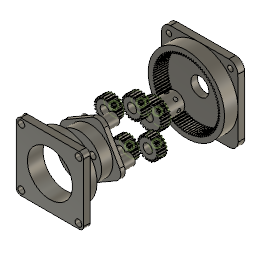
Planetary gear box (simple) (Autodesk Fusion 360 design; units mm, degrees)
part number: 2026-04-07-13-28-31-820
part number: 2026-04-07-13-34-58-780
part number: 2026-04-07-13-35-47-978
part number: 2026-04-07-13-42-23-134
description: Spur Gear; Module: 2.0; Num Teeth: 22; Pressure Angle: 20.0; Backlash: 0.00 mm
part number: 2026-04-07-13-45-37-239
part number: 2026-04-07-13-52-50-834
description: Spur Gear; Module: 2.0; Num Teeth: 28; Pressure Angle: 20.0; Backlash: 0.00 mm
part number: 2026-04-07-13-54-13-736
description: Spur Gear; Module: 1.6; Num Teeth: 88; Pressure Angle: 20.0; Backlash: 0.00 mm
part number: 2026-04-07-14-14-13-761
part number: 2026-04-07-14-24-32-311
Autodesk Fusion 360 part; units mm, degrees
(part 1 of 15)
sketch "Sketch1" plane through (0, 0, 0) normal (0, 1, 0) x (1, 0, 0)
  line L0 (65, -75) -> (-65, -75)
  line L1 (-75, -65) -> (-75, 65)
  line L2 (-65, 75) -> (65, 75)
  line L3 (75, 65) -> (75, -65)
  line L4 (75, -75) -> (-75, 75) construction
  line L5 (-75, -75) -> (75, 75) construction
  circle A0 centre (0, 0) radius 50
  circle A1 centre (63.6396, -63.6396) radius 7.5
  circle A2 centre (-63.6396, -63.6396) radius 7.5
  circle A3 centre (-63.6396, 63.6396) radius 7.5
  circle A4 centre (63.6396, 63.6396) radius 7.5
  arc A5 (65, -75) -> (75, -65) centre (65, -65) ccw
  arc A6 (-75, -65) -> (-65, -75) centre (-65, -65) ccw
  arc A7 (-65, 75) -> (-75, 65) centre (-65, 65) ccw
  arc A8 (75, 65) -> (65, 75) centre (65, 65) ccw
  dimension "d1" = 150
  dimension "d2" = 150
  dimension "d3" = 100
  dimension "d4" = 15
  dimension "d5" = 90
  dimension "d6" = 15
  dimension "d7" = 90
  dimension "d8" = 15
  dimension "d9" = 15
  dimension "d10" = 90
  dimension "d11" = 90
  dimension "d12" = 10
  constraint horizontal L0
  constraint perpendicular L0 L1
  constraint parallel L0 L2
  constraint parallel L1 L3
  constraint coincident L4 A0.centre
  constraint coincident L5 A0.centre
  constraint coincident A0.centre origin
  constraint coincident L4 A1.centre
  constraint coincident L5 A2.centre
  constraint coincident L4 A3.centre
  constraint coincident L5 A4.centre
  constraint coincident L4.start L3
  constraint coincident L4.start L0
  constraint tangent L3 A5
  constraint tangent L0 A5
  constraint coincident L5.start L0
  constraint coincident L5.start L1
  constraint tangent L0 A6
  constraint tangent L1 A6
  constraint equal A5 A6
  constraint coincident L4.end L2
  constraint coincident L4.end L1
  constraint tangent L2 A7
  constraint tangent L1 A7
  constraint equal A5 A7
  constraint coincident L5.end L2
  constraint coincident L5.end L3
  constraint tangent L2 A8
  constraint tangent L3 A8
  constraint equal A5 A8
  measures "d1" distance of L4.end L5.end
  measures "d2" distance of L5.start L4.end
  measures "d3" diameter of A0
  measures "d4" diameter of A1
  measures "d5" distance of A0.centre A1.centre
  measures "d6" diameter of A2
  measures "d7" distance of A0.centre A2.centre
  measures "d8" diameter of A4
  measures "d9" diameter of A3
  measures "d10" distance of A0.centre A4.centre
  measures "d11" distance of A0.centre A3.centre
  measures "d12" radius of A5
extrude "Extrude1" add sketch "Sketch1" along normal blind 15 makes body 1
sketch "Sketch2" plane through (0, 15, 0) normal (0, 1, 0) x (-1, 0, 0)
  circle A0 centre (0, 0) radius 50
  circle A1 centre (63.6396, -63.6396) radius 7.5
  circle A2 centre (-63.6396, 63.6396) radius 7.5
  circle A3 centre (-63.6396, -63.6396) radius 7.5
  circle A4 centre (63.6396, 63.6396) radius 7.5
  arc A5 (-65, 75) -> (-75, 65) centre (-65, 65) ccw
  line L0 (-75, 65) -> (-75, -65)
  arc A6 (-75, -65) -> (-65, -75) centre (-65, -65) ccw
  line L1 (-65, -75) -> (65, -75)
  arc A7 (65, -75) -> (75, -65) centre (65, -65) ccw
  line L2 (75, -65) -> (75, 65)
  arc A8 (75, 65) -> (65, 75) centre (65, 65) ccw
  line L3 (65, 75) -> (-65, 75)
  circle A9 centre (0, 0) radius 70
  dimension "d15" = 140
  constraint coincident A0.centre A9.centre
  measures "d15" diameter of A9
extrude "Extrude2" add sketch "Sketch2" along normal blind 20 contours A9 bodies 1
ref_plane "WorkPlane1" through (0, 65, 0) normal (0, 1, 0) x (-1, 0, 0)
copy_body "Body->Comp1" bodies 1 removing the originals makes body 2 in component "Component"
sketch "Sketch1 (2)" plane through (0, 65, 0) normal (0, 1, 0) x (1, 0, 0) in component "planet gear holder"
  circle A0 centre (0, 0) radius 50
  circle A1 centre (0, 0) radius 50
  line L0 (35, 55) -> (-35, 55)
  line L1 (-55, 35) -> (-55, -35)
  line L2 (-35, -55) -> (35, -55)
  line L3 (55, -35) -> (55, 35)
  line L4 (55, 55) -> (-55, -55) construction
  line L5 (-55, 55) -> (55, -55) construction
  line L6 (0, -50) -> (0, 50) construction
  circle A2 centre (0, -35) radius 7.5
  circle A3 centre (35, 0) radius 7.5
  circle A4 centre (0, 35) radius 7.5
  circle A5 centre (-35, 0) radius 7.5
  arc A6 (35, -55) -> (55, -35) centre (35, -35) ccw
  arc A7 (55, 35) -> (35, 55) centre (35, 35) ccw
  arc A8 (-35, 55) -> (-55, 35) centre (-35, 35) ccw
  arc A9 (-55, -35) -> (-35, -55) centre (-35, -35) ccw
  circle A10 centre (35, -35) radius 12.5
  circle A11 centre (-35, -35) radius 12.5
  circle A12 centre (35, 35) radius 12.5
  circle A13 centre (-35, 35) radius 12.5
  dimension "d19" = 110
  dimension "d20" = 110
  dimension "d21" = 15
  dimension "d22" = 35
  dimension "d24" = 360
  dimension "d25" = 20
  dimension "d28" = 25
  dimension "d29" = 25
  dimension "d30" = 25
  dimension "d31" = 25
  constraint concentric A0 A1
  constraint horizontal L0
  constraint perpendicular L0 L1
  constraint parallel L0 L2
  constraint parallel L1 L3
  constraint coincident L4 A0.centre
  constraint coincident L5 A0.centre
  constraint coincident A0.centre A1.centre
  constraint coincident A0 L6.start
  constraint coincident A1 L6.end
  constraint vertical L6
  constraint coincident L6 A2.centre
  constraint coincident L5.end L2
  constraint coincident L5.end L3
  constraint tangent L2 A6
  constraint tangent L3 A6
  constraint coincident L4.start L3
  constraint coincident L4.start L0
  constraint tangent L3 A7
  constraint tangent L0 A7
  constraint equal A6 A7
  constraint coincident L5.start L0
  constraint coincident L5.start L1
  constraint tangent L0 A8
  constraint tangent L1 A8
  constraint equal A6 A8
  constraint coincident L4.end L2
  constraint coincident L4.end L1
  constraint tangent L2 A9
  constraint tangent L1 A9
  constraint equal A6 A9
  constraint concentric A6 A10
  constraint concentric A9 A11
  constraint concentric A7 A12
  constraint concentric A8 A13
  measures "d19" distance of L4.end L5.end
  measures "d20" distance of L5.start L4.end
  measures "d21" diameter of A2
  measures "d22" distance of A0.centre A2.centre
  measures "d25" radius of A6
  measures "d28" diameter of A10
  measures "d29" diameter of A11
  measures "d30" diameter of A12
  measures "d31" diameter of A13
extrude "Extrude1'" add sketch "Sketch1 (2)" against normal blind 25 separate body contours A0 A1 A10 A11 A12 A13 | A0 A1 A12 | A0 A1 A10 | A0 A1 A13 | A0 A1 A11 picked at (29.7361, 35.2337) picked at (29.7361, -35.2337) picked at (-35.4165, 29.6761) picked at (-35.4165, -29.6761) makes body 3 in component "planet gear holder"
extrude "Extrude2'" add sketch "Sketch1 (2)" along normal blind 40 separate body contours A0 A1 A12 | A0 A1 A12 | A0 A1 A10 | A0 A1 A10 | A0 A1 A13 | A0 A1 A13 | A0 A1 A11 | A0 A1 A11 makes body 4 at (47.4379, 91.6667, -36.2446) makes body 5 at (-22.5621, 91.6667, -36.2446) makes body 6 at (47.4379, 91.6667, 33.7554) makes body 7 at (-22.5621, 78.3333, 36.2446) in component "planet gear holder"
extrude "Extrude3" add sketch "Sketch1 (2)" along normal blind 10 contours A0 A1 A10 A11 A12 A13 | L0 L1 L2 L3 A6 A7 A8 A9 bodies 3 4 5 6 7 in component "planet gear holder"
sketch "Base Circle" plane through (0, 0, 0) normal (0, 0, 1) x (1, 0, 0) in component "Spur Gear 22 teeth"
  circle A0 centre (0, 0) radius 19.686
  circle A1 centre (0, 0) radius 10
extrude "Extrude1''" add sketch "Base Circle" along normal blind 20 separate body makes body 8 in component "Spur Gear 22 teeth"
sketch "Gear Tooth" plane through (0, 0, 0) normal (0, 0, 1) x (1, 0, 0) in component "Spur Gear 22 teeth"
  spline S0 degree 5 poles (20.5963, -1.782) (20.606, -1.7828) (20.6255, -1.7842) (20.6547, -1.7856) (20.6937, -1.7861) (20.7426, -1.7846) (20.7915, -1.7818) (20.8404, -1.7781) (20.8894, -1.7739) (20.9384, -1.7693) (20.9874, -1.7645) (21.0364, -1.7592) (21.0854, -1.7533) (21.1344, -1.7468) (21.1835, -1.7395) (21.2325, -1.7317) (21.2815, -1.7232) (21.3306, -1.7143) (21.3796, -1.705) (21.4286, -1.6954) (21.4776, -1.6853) (21.5266, -1.6749) (21.5756, -1.6641) (21.6246, -1.6528) (21.6736, -1.6411) (21.7225, -1.629) (21.7714, -1.6165) (21.8204, -1.6036) (21.8693, -1.5904) (21.9182, -1.5768) (21.967, -1.5629) (22.0159, -1.5487) (22.0647, -1.5341) (22.1135, -1.5191) (22.1622, -1.5038) (22.211, -1.4882) (22.2597, -1.4723) (22.3084, -1.456) (22.3571, -1.4394) (22.4057, -1.4225) (22.4543, -1.4053) (22.5029, -1.3878) (22.5514, -1.37) (22.6, -1.3519) (22.6484, -1.3335) (22.6969, -1.3148) (22.7453, -1.2958) (22.7937, -1.2765) (22.842, -1.2569) (22.8903, -1.237) (22.9386, -1.2169) (22.9868, -1.1964) (23.035, -1.1757) (23.0832, -1.1548) (23.1313, -1.1335) (23.1794, -1.112) (23.2274, -1.0902) (23.2754, -1.0681) (23.3233, -1.0457) (23.3712, -1.0231) (23.4191, -1.0003) (23.4669, -0.9772) (23.5146, -0.9538) (23.5624, -0.9301) (23.61, -0.9062) (23.6577, -0.8821) (23.7052, -0.8577) (23.7528, -0.833) (23.8002, -0.8081) (23.8477, -0.7829) (23.895, -0.7575) (23.9329, -0.737) (23.9613, -0.7215) (23.9802, -0.7111) (23.9896, -0.7059) knots 0 0 0 0 0 0 0.01428571 0.02857143 0.04285714 0.05714286 0.07142857 0.08571429 0.1 0.11428571 0.12857143 0.14285714 0.15714286 0.17142857 0.18571429 0.2 0.21428571 0.22857143 0.24285714 0.25714286 0.27142857 0.28571429 0.3 0.31428571 0.32857143 0.34285714 0.35714286 0.37142857 0.38571429 0.4 0.41428571 0.42857143 0.44285714 0.45714286 0.47142857 0.48571429 0.5 0.51428571 0.52857143 0.54285714 0.55714286 0.57142857 0.58571429 0.6 0.61428571 0.62857143 0.64285714 0.65714286 0.67142857 0.68571429 0.7 0.71428571 0.72857143 0.74285714 0.75714286 0.77142857 0.78571429 0.8 0.81428571 0.82857143 0.84285714 0.85714286 0.87142857 0.88571429 0.9 0.91428571 0.92857143 0.94285714 0.95714286 0.97142857 0.98571429 1 1 1 1 1 1
  spline S1 degree 5 poles (20.5963, 1.782) (20.606, 1.7828) (20.6255, 1.7842) (20.6547, 1.7856) (20.6937, 1.7861) (20.7426, 1.7846) (20.7915, 1.7818) (20.8404, 1.7781) (20.8894, 1.7739) (20.9384, 1.7693) (20.9874, 1.7645) (21.0364, 1.7592) (21.0854, 1.7533) (21.1344, 1.7468) (21.1835, 1.7395) (21.2325, 1.7317) (21.2815, 1.7232) (21.3306, 1.7143) (21.3796, 1.705) (21.4286, 1.6954) (21.4776, 1.6853) (21.5266, 1.6749) (21.5756, 1.6641) (21.6246, 1.6528) (21.6736, 1.6411) (21.7225, 1.629) (21.7714, 1.6165) (21.8204, 1.6036) (21.8693, 1.5904) (21.9182, 1.5768) (21.967, 1.5629) (22.0159, 1.5487) (22.0647, 1.5341) (22.1135, 1.5191) (22.1622, 1.5038) (22.211, 1.4882) (22.2597, 1.4723) (22.3084, 1.456) (22.3571, 1.4394) (22.4057, 1.4225) (22.4543, 1.4053) (22.5029, 1.3878) (22.5514, 1.37) (22.6, 1.3519) (22.6484, 1.3335) (22.6969, 1.3148) (22.7453, 1.2958) (22.7937, 1.2765) (22.842, 1.2569) (22.8903, 1.237) (22.9386, 1.2169) (22.9868, 1.1964) (23.035, 1.1757) (23.0832, 1.1548) (23.1313, 1.1335) (23.1794, 1.112) (23.2274, 1.0902) (23.2754, 1.0681) (23.3233, 1.0457) (23.3712, 1.0231) (23.4191, 1.0003) (23.4669, 0.9772) (23.5146, 0.9538) (23.5624, 0.9301) (23.61, 0.9062) (23.6577, 0.8821) (23.7052, 0.8577) (23.7528, 0.833) (23.8002, 0.8081) (23.8477, 0.7829) (23.895, 0.7575) (23.9329, 0.737) (23.9613, 0.7215) (23.9802, 0.7111) (23.9896, 0.7059) knots 0 0 0 0 0 0 0.01428571 0.02857143 0.04285714 0.05714286 0.07142857 0.08571429 0.1 0.11428571 0.12857143 0.14285714 0.15714286 0.17142857 0.18571429 0.2 0.21428571 0.22857143 0.24285714 0.25714286 0.27142857 0.28571429 0.3 0.31428571 0.32857143 0.34285714 0.35714286 0.37142857 0.38571429 0.4 0.41428571 0.42857143 0.44285714 0.45714286 0.47142857 0.48571429 0.5 0.51428571 0.52857143 0.54285714 0.55714286 0.57142857 0.58571429 0.6 0.61428571 0.62857143 0.64285714 0.65714286 0.67142857 0.68571429 0.7 0.71428571 0.72857143 0.74285714 0.75714286 0.77142857 0.78571429 0.8 0.81428571 0.82857143 0.84285714 0.85714286 0.87142857 0.88571429 0.9 0.91428571 0.92857143 0.94285714 0.95714286 0.97142857 0.98571429 1 1 1 1 1 1
  arc A0 (23.9896, -0.7059) -> (23.9896, 0.7059) centre (0, 0) ccw
  line L0 (19.6028, -1.696) -> (20.5963, -1.782)
  line L1 (19.6028, 1.696) -> (20.5963, 1.782)
  line L2 (19.6028, -1.696) -> (19.6028, 1.696)
  point P0 (20.8351, -1.7784)
  point P1 (21.0756, -1.7544)
  point P2 (21.3171, -1.7167)
  point P3 (21.5593, -1.6676)
  point P4 (21.8021, -1.6084)
  point P5 (22.0453, -1.5398)
  point P6 (22.2887, -1.4626)
  point P7 (22.5322, -1.377)
  point P8 (22.7757, -1.2836)
  point P9 (23.0191, -1.1825)
  point P10 (23.2623, -1.074)
  point P11 (23.5052, -0.9583)
  point P12 (23.7477, -0.8356)
  point P13 (20.8351, 1.7784)
  point P14 (21.0756, 1.7544)
  point P15 (21.3171, 1.7167)
  point P16 (21.5593, 1.6676)
  point P17 (21.8021, 1.6084)
  point P18 (22.0453, 1.5398)
  point P19 (22.2887, 1.4626)
  point P20 (22.5322, 1.377)
  point P21 (22.7757, 1.2836)
  point P22 (23.0191, 1.1825)
  point P23 (23.2623, 1.074)
  point P24 (23.5052, 0.9583)
  point P25 (23.7477, 0.8356)
extrude "Extrude2''" add sketch "Gear Tooth" along normal blind 20 bodies 8 in component "Spur Gear 22 teeth"
pattern_circular "C-Pattern1" count 22 over 360 about axis through (0, 0, 0) along (0, 0, 1) of "Extrude2''" in component "Spur Gear 22 teeth"
sketch "Diametrial Pitch Circle" plane through (0, 0, 0) normal (0, 0, 1) x (1, 0, 0) in component "Spur Gear 22 teeth"
  circle A0 centre (0, 0) radius 22 construction
sketch "Base Circle (2)" plane through (0, 0, 0) normal (0, 0, 1) x (1, 0, 0) in component "Spur Gear 28 teeth"
  circle A0 centre (0, 0) radius 25.686
  circle A1 centre (0, 0) radius 10
extrude "Extrude1'''" add sketch "Base Circle (2)" along normal blind 20 separate body makes body 9 in component "Spur Gear 28 teeth"
sketch "Gear Tooth (2)" plane through (0, 0, 0) normal (0, 0, 1) x (1, 0, 0) in component "Spur Gear 28 teeth"
  spline S0 degree 5 poles (26.2451, -1.8667) (26.2559, -1.8674) (26.2774, -1.8687) (26.3098, -1.8698) (26.3529, -1.8699) (26.4069, -1.8679) (26.461, -1.8644) (26.515, -1.8601) (26.5691, -1.8552) (26.6232, -1.8501) (26.6773, -1.8446) (26.7314, -1.8386) (26.7855, -1.8321) (26.8396, -1.8248) (26.8937, -1.8169) (26.9478, -1.8082) (27.0019, -1.7991) (27.056, -1.7894) (27.1101, -1.7794) (27.1642, -1.7689) (27.2182, -1.7581) (27.2723, -1.7469) (27.3263, -1.7352) (27.3803, -1.7231) (27.4343, -1.7106) (27.4883, -1.6977) (27.5423, -1.6844) (27.5962, -1.6707) (27.6502, -1.6566) (27.7041, -1.6422) (27.7579, -1.6274) (27.8118, -1.6123) (27.8656, -1.5968) (27.9194, -1.581) (27.9732, -1.5648) (28.027, -1.5483) (28.0807, -1.5315) (28.1344, -1.5143) (28.1881, -1.4969) (28.2417, -1.4791) (28.2953, -1.461) (28.3489, -1.4425) (28.4025, -1.4238) (28.456, -1.4048) (28.5095, -1.3854) (28.5629, -1.3658) (28.6163, -1.3459) (28.6697, -1.3256) (28.7231, -1.3051) (28.7764, -1.2843) (28.8296, -1.2632) (28.8829, -1.2418) (28.9361, -1.2202) (28.9892, -1.1983) (29.0423, -1.176) (29.0954, -1.1536) (29.1485, -1.1308) (29.2015, -1.1078) (29.2544, -1.0845) (29.3073, -1.0609) (29.3602, -1.0371) (29.413, -1.013) (29.4658, -0.9886) (29.5186, -0.964) (29.5712, -0.9391) (29.6239, -0.914) (29.6765, -0.8886) (29.729, -0.863) (29.7816, -0.8371) (29.834, -0.8109) (29.8864, -0.7845) (29.9283, -0.7632) (29.9597, -0.7471) (29.9806, -0.7364) (29.9911, -0.731) knots 0 0 0 0 0 0 0.01428571 0.02857143 0.04285714 0.05714286 0.07142857 0.08571429 0.1 0.11428571 0.12857143 0.14285714 0.15714286 0.17142857 0.18571429 0.2 0.21428571 0.22857143 0.24285714 0.25714286 0.27142857 0.28571429 0.3 0.31428571 0.32857143 0.34285714 0.35714286 0.37142857 0.38571429 0.4 0.41428571 0.42857143 0.44285714 0.45714286 0.47142857 0.48571429 0.5 0.51428571 0.52857143 0.54285714 0.55714286 0.57142857 0.58571429 0.6 0.61428571 0.62857143 0.64285714 0.65714286 0.67142857 0.68571429 0.7 0.71428571 0.72857143 0.74285714 0.75714286 0.77142857 0.78571429 0.8 0.81428571 0.82857143 0.84285714 0.85714286 0.87142857 0.88571429 0.9 0.91428571 0.92857143 0.94285714 0.95714286 0.97142857 0.98571429 1 1 1 1 1 1
  spline S1 degree 5 poles (26.2451, 1.8667) (26.2559, 1.8674) (26.2774, 1.8687) (26.3098, 1.8698) (26.3529, 1.8699) (26.4069, 1.8679) (26.461, 1.8644) (26.515, 1.8601) (26.5691, 1.8552) (26.6232, 1.8501) (26.6773, 1.8446) (26.7314, 1.8386) (26.7855, 1.8321) (26.8396, 1.8248) (26.8937, 1.8169) (26.9478, 1.8082) (27.0019, 1.7991) (27.056, 1.7894) (27.1101, 1.7794) (27.1642, 1.7689) (27.2182, 1.7581) (27.2723, 1.7469) (27.3263, 1.7352) (27.3803, 1.7231) (27.4343, 1.7106) (27.4883, 1.6977) (27.5423, 1.6844) (27.5962, 1.6707) (27.6502, 1.6566) (27.7041, 1.6422) (27.7579, 1.6274) (27.8118, 1.6123) (27.8656, 1.5968) (27.9194, 1.581) (27.9732, 1.5648) (28.027, 1.5483) (28.0807, 1.5315) (28.1344, 1.5143) (28.1881, 1.4969) (28.2417, 1.4791) (28.2953, 1.461) (28.3489, 1.4425) (28.4025, 1.4238) (28.456, 1.4048) (28.5095, 1.3854) (28.5629, 1.3658) (28.6163, 1.3459) (28.6697, 1.3256) (28.7231, 1.3051) (28.7764, 1.2843) (28.8296, 1.2632) (28.8829, 1.2418) (28.9361, 1.2202) (28.9892, 1.1983) (29.0423, 1.176) (29.0954, 1.1536) (29.1485, 1.1308) (29.2015, 1.1078) (29.2544, 1.0845) (29.3073, 1.0609) (29.3602, 1.0371) (29.413, 1.013) (29.4658, 0.9886) (29.5186, 0.964) (29.5712, 0.9391) (29.6239, 0.914) (29.6765, 0.8886) (29.729, 0.863) (29.7816, 0.8371) (29.834, 0.8109) (29.8864, 0.7845) (29.9283, 0.7632) (29.9597, 0.7471) (29.9806, 0.7364) (29.9911, 0.731) knots 0 0 0 0 0 0 0.01428571 0.02857143 0.04285714 0.05714286 0.07142857 0.08571429 0.1 0.11428571 0.12857143 0.14285714 0.15714286 0.17142857 0.18571429 0.2 0.21428571 0.22857143 0.24285714 0.25714286 0.27142857 0.28571429 0.3 0.31428571 0.32857143 0.34285714 0.35714286 0.37142857 0.38571429 0.4 0.41428571 0.42857143 0.44285714 0.45714286 0.47142857 0.48571429 0.5 0.51428571 0.52857143 0.54285714 0.55714286 0.57142857 0.58571429 0.6 0.61428571 0.62857143 0.64285714 0.65714286 0.67142857 0.68571429 0.7 0.71428571 0.72857143 0.74285714 0.75714286 0.77142857 0.78571429 0.8 0.81428571 0.82857143 0.84285714 0.85714286 0.87142857 0.88571429 0.9 0.91428571 0.92857143 0.94285714 0.95714286 0.97142857 0.98571429 1 1 1 1 1 1
  arc A0 (29.9911, -0.731) -> (29.9911, 0.731) centre (0, 0) ccw
  line L0 (25.6113, -1.8216) -> (26.2451, -1.8667)
  line L1 (25.6113, 1.8216) -> (26.2451, 1.8667)
  line L2 (25.6113, -1.8216) -> (25.6113, 1.8216)
  point P0 (26.5097, -1.8604)
  point P1 (26.7757, -1.8331)
  point P2 (27.0425, -1.7918)
  point P3 (27.31, -1.7387)
  point P4 (27.5779, -1.6753)
  point P5 (27.8462, -1.6024)
  point P6 (28.1146, -1.5206)
  point P7 (28.3831, -1.4305)
  point P8 (28.6517, -1.3324)
  point P9 (28.9201, -1.2266)
  point P10 (29.1884, -1.1134)
  point P11 (29.4563, -0.9929)
  point P12 (29.7239, -0.8654)
  point P13 (26.5097, 1.8604)
  point P14 (26.7757, 1.8331)
  point P15 (27.0425, 1.7918)
  point P16 (27.31, 1.7387)
  point P17 (27.5779, 1.6753)
  point P18 (27.8462, 1.6024)
  point P19 (28.1146, 1.5206)
  point P20 (28.3831, 1.4305)
  point P21 (28.6517, 1.3324)
  point P22 (28.9201, 1.2266)
  point P23 (29.1884, 1.1134)
  point P24 (29.4563, 0.9929)
  point P25 (29.7239, 0.8654)
extrude "Extrude2'''" add sketch "Gear Tooth (2)" along normal blind 20 bodies 9 in component "Spur Gear 28 teeth"
pattern_circular "C-Pattern1'" count 28 over 360 about axis through (0, 0, 0) along (0, 0, 1) of "Extrude2'''" in component "Spur Gear 28 teeth"
sketch "Diametrial Pitch Circle (2)" plane through (0, 0, 0) normal (0, 0, 1) x (1, 0, 0) in component "Spur Gear 28 teeth"
  circle A0 centre (0, 0) radius 28 construction
sketch "Sketch4" plane through (0, 0, 0) normal (0, 0, -1) x (1, 0, 0) in component "Spur Gear 28 teeth"
  circle A0 centre (0, 0) radius 10
  arc A1 (24.5734, 7.4779) -> (23.8746, 9.4748) centre (0, 0) ccw
  line L0 (23.8746, 9.4748) -> (24.4559, 9.7055)
  spline S0 degree 5 poles (24.4559, 9.7055) (24.466, 9.7095) (24.4859, 9.7177) (24.5156, 9.7307) (24.5545, 9.7494) (24.6023, 9.7746) (24.6494, 9.8012) (24.6963, 9.8286) (24.7429, 9.8564) (24.7894, 9.8845) (24.8357, 9.9129) (24.8819, 9.9418) (24.9278, 9.9712) (24.9734, 10.0012) (25.0187, 10.0318) (25.0637, 10.0631) (25.1085, 10.0948) (25.153, 10.127) (25.1974, 10.1595) (25.2416, 10.1924) (25.2856, 10.2256) (25.3294, 10.2591) (25.3731, 10.2931) (25.4165, 10.3274) (25.4597, 10.3621) (25.5027, 10.3972) (25.5456, 10.4326) (25.5882, 10.4683) (25.6307, 10.5044) (25.673, 10.5408) (25.7151, 10.5775) (25.7571, 10.6145) (25.7989, 10.6518) (25.8405, 10.6894) (25.882, 10.7273) (25.9232, 10.7654) (25.9643, 10.8039) (26.0053, 10.8427) (26.0461, 10.8817) (26.0867, 10.921) (26.1271, 10.9606) (26.1674, 11.0004) (26.2075, 11.0406) (26.2475, 11.0809) (26.2873, 11.1216) (26.3269, 11.1624) (26.3664, 11.2036) (26.4057, 11.245) (26.4449, 11.2866) (26.4839, 11.3285) (26.5227, 11.3706) (26.5614, 11.4129) (26.5999, 11.4555) (26.6383, 11.4984) (26.6765, 11.5414) (26.7146, 11.5847) (26.7525, 11.6282) (26.7902, 11.672) (26.8279, 11.716) (26.8653, 11.7601) (26.9026, 11.8046) (26.9397, 11.8492) (26.9767, 11.894) (27.0136, 11.9391) (27.0502, 11.9844) (27.0868, 12.0299) (27.1231, 12.0755) (27.1594, 12.1215) (27.1954, 12.1676) (27.2314, 12.2139) (27.2671, 12.2604) (27.2956, 12.2978) (27.3169, 12.3259) (27.3311, 12.3447) (27.3382, 12.3541) knots 0 0 0 0 0 0 0.01428571 0.02857143 0.04285714 0.05714286 0.07142857 0.08571429 0.1 0.11428571 0.12857143 0.14285714 0.15714286 0.17142857 0.18571429 0.2 0.21428571 0.22857143 0.24285714 0.25714286 0.27142857 0.28571429 0.3 0.31428571 0.32857143 0.34285714 0.35714286 0.37142857 0.38571429 0.4 0.41428571 0.42857143 0.44285714 0.45714286 0.47142857 0.48571429 0.5 0.51428571 0.52857143 0.54285714 0.55714286 0.57142857 0.58571429 0.6 0.61428571 0.62857143 0.64285714 0.65714286 0.67142857 0.68571429 0.7 0.71428571 0.72857143 0.74285714 0.75714286 0.77142857 0.78571429 0.8 0.81428571 0.82857143 0.84285714 0.85714286 0.87142857 0.88571429 0.9 0.91428571 0.92857143 0.94285714 0.95714286 0.97142857 0.98571429 1 1 1 1 1 1
  arc A2 (27.3382, 12.3541) -> (26.7039, 13.6712) centre (0, 0) ccw
  spline S1 degree 5 poles (22.8361, 13.0691) (22.8455, 13.0745) (22.8643, 13.085) (22.893, 13.1) (22.9319, 13.1188) (22.9814, 13.1404) (23.0315, 13.1608) (23.0821, 13.1803) (23.133, 13.1994) (23.1839, 13.2182) (23.2351, 13.2367) (23.2864, 13.2548) (23.338, 13.2724) (23.3899, 13.2894) (23.4421, 13.3057) (23.4946, 13.3214) (23.5473, 13.3366) (23.6002, 13.3514) (23.6533, 13.3658) (23.7066, 13.3798) (23.76, 13.3935) (23.8135, 13.4069) (23.8673, 13.4198) (23.9212, 13.4324) (23.9753, 13.4445) (24.0295, 13.4563) (24.0839, 13.4677) (24.1385, 13.4788) (24.1932, 13.4895) (24.248, 13.4999) (24.3029, 13.51) (24.358, 13.5197) (24.4132, 13.5291) (24.4686, 13.5382) (24.524, 13.547) (24.5796, 13.5555) (24.6353, 13.5636) (24.6912, 13.5714) (24.7471, 13.579) (24.8032, 13.5862) (24.8593, 13.5932) (24.9156, 13.5998) (24.972, 13.6062) (25.0284, 13.6123) (25.085, 13.618) (25.1417, 13.6235) (25.1985, 13.6288) (25.2553, 13.6337) (25.3123, 13.6383) (25.3694, 13.6427) (25.4265, 13.6468) (25.4838, 13.6507) (25.5411, 13.6542) (25.5985, 13.6575) (25.656, 13.6606) (25.7136, 13.6633) (25.7712, 13.6659) (25.829, 13.6681) (25.8868, 13.6701) (25.9447, 13.6718) (26.0027, 13.6733) (26.0607, 13.6745) (26.1188, 13.6754) (26.177, 13.6761) (26.2353, 13.6766) (26.2936, 13.6768) (26.3521, 13.6767) (26.4105, 13.6765) (26.4691, 13.6759) (26.5277, 13.6751) (26.5863, 13.6741) (26.6333, 13.6731) (26.6686, 13.6722) (26.6921, 13.6715) (26.7039, 13.6712) knots 0 0 0 0 0 0 0.01428571 0.02857143 0.04285714 0.05714286 0.07142857 0.08571429 0.1 0.11428571 0.12857143 0.14285714 0.15714286 0.17142857 0.18571429 0.2 0.21428571 0.22857143 0.24285714 0.25714286 0.27142857 0.28571429 0.3 0.31428571 0.32857143 0.34285714 0.35714286 0.37142857 0.38571429 0.4 0.41428571 0.42857143 0.44285714 0.45714286 0.47142857 0.48571429 0.5 0.51428571 0.52857143 0.54285714 0.55714286 0.57142857 0.58571429 0.6 0.61428571 0.62857143 0.64285714 0.65714286 0.67142857 0.68571429 0.7 0.71428571 0.72857143 0.74285714 0.75714286 0.77142857 0.78571429 0.8 0.81428571 0.82857143 0.84285714 0.85714286 0.87142857 0.88571429 0.9 0.91428571 0.92857143 0.94285714 0.95714286 0.97142857 0.98571429 1 1 1 1 1 1
  line L1 (22.8361, 13.0691) -> (22.2933, 12.7585)
  arc A3 (22.2933, 12.7585) -> (21.1677, 14.5499) centre (0, 0) ccw
  line L2 (21.1677, 14.5499) -> (21.6831, 14.9041)
  spline S2 degree 5 poles (21.6831, 14.9041) (21.692, 14.9103) (21.7096, 14.9227) (21.7356, 14.942) (21.7694, 14.9689) (21.8104, 15.0041) (21.8505, 15.0405) (21.89, 15.0776) (21.9293, 15.1151) (21.9683, 15.1528) (22.0072, 15.1909) (22.0458, 15.2293) (22.084, 15.2681) (22.1218, 15.3075) (22.1592, 15.3475) (22.1961, 15.388) (22.2327, 15.4289) (22.2689, 15.4701) (22.3049, 15.5117) (22.3407, 15.5536) (22.3762, 15.5958) (22.4115, 15.6382) (22.4465, 15.681) (22.4812, 15.7242) (22.5156, 15.7676) (22.5497, 15.8114) (22.5836, 15.8554) (22.6172, 15.8998) (22.6506, 15.9444) (22.6838, 15.9893) (22.7167, 16.0344) (22.7494, 16.0798) (22.7818, 16.1255) (22.814, 16.1714) (22.846, 16.2176) (22.8777, 16.264) (22.9093, 16.3107) (22.9405, 16.3576) (22.9716, 16.4047) (23.0025, 16.452) (23.0331, 16.4996) (23.0635, 16.5474) (23.0937, 16.5955) (23.1237, 16.6437) (23.1534, 16.6922) (23.183, 16.7409) (23.2123, 16.7897) (23.2414, 16.8388) (23.2703, 16.8881) (23.299, 16.9377) (23.3275, 16.9874) (23.3558, 17.0373) (23.3839, 17.0874) (23.4118, 17.1377) (23.4395, 17.1881) (23.467, 17.2388) (23.4942, 17.2897) (23.5213, 17.3407) (23.5482, 17.392) (23.5749, 17.4434) (23.6013, 17.495) (23.6276, 17.5468) (23.6537, 17.5987) (23.6796, 17.6508) (23.7053, 17.7031) (23.7308, 17.7556) (23.7561, 17.8083) (23.7812, 17.8611) (23.8061, 17.9141) (23.8308, 17.9672) (23.8553, 18.0205) (23.8748, 18.0633) (23.8893, 18.0954) (23.8989, 18.1169) (23.9037, 18.1277) knots 0 0 0 0 0 0 0.01428571 0.02857143 0.04285714 0.05714286 0.07142857 0.08571429 0.1 0.11428571 0.12857143 0.14285714 0.15714286 0.17142857 0.18571429 0.2 0.21428571 0.22857143 0.24285714 0.25714286 0.27142857 0.28571429 0.3 0.31428571 0.32857143 0.34285714 0.35714286 0.37142857 0.38571429 0.4 0.41428571 0.42857143 0.44285714 0.45714286 0.47142857 0.48571429 0.5 0.51428571 0.52857143 0.54285714 0.55714286 0.57142857 0.58571429 0.6 0.61428571 0.62857143 0.64285714 0.65714286 0.67142857 0.68571429 0.7 0.71428571 0.72857143 0.74285714 0.75714286 0.77142857 0.78571429 0.8 0.81428571 0.82857143 0.84285714 0.85714286 0.87142857 0.88571429 0.9 0.91428571 0.92857143 0.94285714 0.95714286 0.97142857 0.98571429 1 1 1 1 1 1
  arc A4 (23.9037, 18.1277) -> (22.9922, 19.2706) centre (0, 0) ccw
  spline S3 degree 5 poles (19.3554, 17.823) (19.3633, 17.8303) (19.3794, 17.8447) (19.404, 17.8658) (19.4377, 17.8927) (19.4812, 17.9248) (19.5255, 17.9558) (19.5705, 17.9861) (19.6158, 18.016) (19.6613, 18.0457) (19.7071, 18.0752) (19.7531, 18.1042) (19.7995, 18.1329) (19.8463, 18.1609) (19.8936, 18.1884) (19.9412, 18.2154) (19.9893, 18.242) (20.0376, 18.2682) (20.0861, 18.294) (20.1349, 18.3196) (20.1839, 18.3448) (20.2332, 18.3698) (20.2827, 18.3943) (20.3324, 18.4186) (20.3825, 18.4425) (20.4327, 18.466) (20.4832, 18.4892) (20.534, 18.5121) (20.5849, 18.5348) (20.636, 18.5571) (20.6874, 18.5792) (20.7389, 18.6009) (20.7906, 18.6224) (20.8426, 18.6436) (20.8947, 18.6645) (20.947, 18.6851) (20.9995, 18.7054) (21.0522, 18.7255) (21.105, 18.7453) (21.1581, 18.7648) (21.2113, 18.7841) (21.2647, 18.8031) (21.3182, 18.8218) (21.3719, 18.8403) (21.4258, 18.8585) (21.4798, 18.8765) (21.534, 18.8942) (21.5884, 18.9117) (21.6429, 18.9289) (21.6975, 18.9459) (21.7523, 18.9626) (21.8073, 18.9791) (21.8624, 18.9953) (21.9176, 19.0113) (21.973, 19.0271) (22.0285, 19.0426) (22.0842, 19.0579) (22.1399, 19.0729) (22.1959, 19.0877) (22.2519, 19.1023) (22.3081, 19.1166) (22.3645, 19.1307) (22.4209, 19.1446) (22.4775, 19.1582) (22.5342, 19.1716) (22.591, 19.1848) (22.648, 19.1977) (22.7051, 19.2104) (22.7623, 19.2229) (22.8196, 19.2352) (22.877, 19.2473) (22.923, 19.2567) (22.9576, 19.2637) (22.9807, 19.2683) (22.9922, 19.2706) knots 0 0 0 0 0 0 0.01428571 0.02857143 0.04285714 0.05714286 0.07142857 0.08571429 0.1 0.11428571 0.12857143 0.14285714 0.15714286 0.17142857 0.18571429 0.2 0.21428571 0.22857143 0.24285714 0.25714286 0.27142857 0.28571429 0.3 0.31428571 0.32857143 0.34285714 0.35714286 0.37142857 0.38571429 0.4 0.41428571 0.42857143 0.44285714 0.45714286 0.47142857 0.48571429 0.5 0.51428571 0.52857143 0.54285714 0.55714286 0.57142857 0.58571429 0.6 0.61428571 0.62857143 0.64285714 0.65714286 0.67142857 0.68571429 0.7 0.71428571 0.72857143 0.74285714 0.75714286 0.77142857 0.78571429 0.8 0.81428571 0.82857143 0.84285714 0.85714286 0.87142857 0.88571429 0.9 0.91428571 0.92857143 0.94285714 0.95714286 0.97142857 0.98571429 1 1 1 1 1 1
  line L3 (19.3554, 17.823) -> (18.8953, 17.3993)
  arc A5 (18.8953, 17.3993) -> (17.3993, 18.8953) centre (0, 0) ccw
  line L4 (17.3993, 18.8953) -> (17.823, 19.3554)
  spline S4 degree 5 poles (17.823, 19.3554) (17.8303, 19.3634) (17.8447, 19.3794) (17.8658, 19.404) (17.8927, 19.4377) (17.9248, 19.4812) (17.9558, 19.5255) (17.9861, 19.5705) (18.016, 19.6158) (18.0457, 19.6613) (18.0752, 19.7071) (18.1042, 19.7531) (18.1329, 19.7995) (18.1609, 19.8463) (18.1884, 19.8936) (18.2154, 19.9412) (18.242, 19.9893) (18.2682, 20.0376) (18.294, 20.0861) (18.3196, 20.1349) (18.3448, 20.1839) (18.3698, 20.2332) (18.3943, 20.2827) (18.4186, 20.3324) (18.4425, 20.3825) (18.466, 20.4327) (18.4892, 20.4832) (18.5121, 20.534) (18.5348, 20.5849) (18.5571, 20.636) (18.5792, 20.6874) (18.6009, 20.7389) (18.6224, 20.7906) (18.6436, 20.8426) (18.6645, 20.8947) (18.6851, 20.947) (18.7054, 20.9995) (18.7255, 21.0522) (18.7453, 21.105) (18.7648, 21.1581) (18.7841, 21.2113) (18.8031, 21.2647) (18.8218, 21.3182) (18.8403, 21.3719) (18.8585, 21.4258) (18.8765, 21.4798) (18.8942, 21.534) (18.9117, 21.5884) (18.9289, 21.6429) (18.9459, 21.6975) (18.9626, 21.7523) (18.9791, 21.8073) (18.9953, 21.8624) (19.0113, 21.9176) (19.0271, 21.973) (19.0426, 22.0285) (19.0579, 22.0842) (19.0729, 22.1399) (19.0877, 22.1959) (19.1023, 22.2519) (19.1166, 22.3081) (19.1307, 22.3645) (19.1446, 22.4209) (19.1582, 22.4775) (19.1716, 22.5342) (19.1848, 22.591) (19.1977, 22.648) (19.2104, 22.7051) (19.2229, 22.7623) (19.2352, 22.8196) (19.2473, 22.877) (19.2567, 22.923) (19.2637, 22.9576) (19.2683, 22.9807) (19.2706, 22.9922) knots 0 0 0 0 0 0 0.01428571 0.02857143 0.04285714 0.05714286 0.07142857 0.08571429 0.1 0.11428571 0.12857143 0.14285714 0.15714286 0.17142857 0.18571429 0.2 0.21428571 0.22857143 0.24285714 0.25714286 0.27142857 0.28571429 0.3 0.31428571 0.32857143 0.34285714 0.35714286 0.37142857 0.38571429 0.4 0.41428571 0.42857143 0.44285714 0.45714286 0.47142857 0.48571429 0.5 0.51428571 0.52857143 0.54285714 0.55714286 0.57142857 0.58571429 0.6 0.61428571 0.62857143 0.64285714 0.65714286 0.67142857 0.68571429 0.7 0.71428571 0.72857143 0.74285714 0.75714286 0.77142857 0.78571429 0.8 0.81428571 0.82857143 0.84285714 0.85714286 0.87142857 0.88571429 0.9 0.91428571 0.92857143 0.94285714 0.95714286 0.97142857 0.98571429 1 1 1 1 1 1
  arc A6 (19.2706, 22.9922) -> (18.1277, 23.9037) centre (0, 0) ccw
  spline S5 degree 5 poles (14.9041, 21.6831) (14.9103, 21.692) (14.9227, 21.7096) (14.942, 21.7356) (14.9689, 21.7694) (15.0041, 21.8104) (15.0405, 21.8505) (15.0776, 21.89) (15.1151, 21.9293) (15.1528, 21.9683) (15.1909, 22.0072) (15.2293, 22.0458) (15.2681, 22.084) (15.3075, 22.1218) (15.3475, 22.1592) (15.388, 22.1961) (15.4289, 22.2327) (15.4701, 22.2689) (15.5117, 22.3049) (15.5536, 22.3407) (15.5958, 22.3762) (15.6382, 22.4115) (15.681, 22.4465) (15.7242, 22.4812) (15.7676, 22.5156) (15.8114, 22.5497) (15.8554, 22.5836) (15.8998, 22.6172) (15.9444, 22.6506) (15.9893, 22.6838) (16.0344, 22.7167) (16.0798, 22.7494) (16.1255, 22.7818) (16.1714, 22.814) (16.2176, 22.846) (16.264, 22.8777) (16.3107, 22.9093) (16.3576, 22.9405) (16.4047, 22.9716) (16.452, 23.0025) (16.4996, 23.0331) (16.5474, 23.0635) (16.5955, 23.0937) (16.6437, 23.1237) (16.6922, 23.1534) (16.7409, 23.183) (16.7897, 23.2123) (16.8388, 23.2414) (16.8881, 23.2703) (16.9377, 23.299) (16.9874, 23.3275) (17.0373, 23.3558) (17.0874, 23.3839) (17.1377, 23.4118) (17.1881, 23.4395) (17.2388, 23.467) (17.2897, 23.4942) (17.3407, 23.5213) (17.392, 23.5482) (17.4434, 23.5749) (17.495, 23.6013) (17.5468, 23.6276) (17.5987, 23.6537) (17.6508, 23.6796) (17.7031, 23.7053) (17.7556, 23.7308) (17.8083, 23.7561) (17.8611, 23.7812) (17.914, 23.8061) (17.9672, 23.8308) (18.0205, 23.8553) (18.0633, 23.8748) (18.0954, 23.8893) (18.1169, 23.8989) (18.1277, 23.9037) knots 0 0 0 0 0 0 0.01428571 0.02857143 0.04285714 0.05714286 0.07142857 0.08571429 0.1 0.11428571 0.12857143 0.14285714 0.15714286 0.17142857 0.18571429 0.2 0.21428571 0.22857143 0.24285714 0.25714286 0.27142857 0.28571429 0.3 0.31428571 0.32857143 0.34285714 0.35714286 0.37142857 0.38571429 0.4 0.41428571 0.42857143 0.44285714 0.45714286 0.47142857 0.48571429 0.5 0.51428571 0.52857143 0.54285714 0.55714286 0.57142857 0.58571429 0.6 0.61428571 0.62857143 0.64285714 0.65714286 0.67142857 0.68571429 0.7 0.71428571 0.72857143 0.74285714 0.75714286 0.77142857 0.78571429 0.8 0.81428571 0.82857143 0.84285714 0.85714286 0.87142857 0.88571429 0.9 0.91428571 0.92857143 0.94285714 0.95714286 0.97142857 0.98571429 1 1 1 1 1 1
  line L5 (14.9041, 21.6831) -> (14.5499, 21.1677)
  arc A7 (14.5499, 21.1677) -> (12.7585, 22.2933) centre (0, 0) ccw
  line L6 (12.7585, 22.2933) -> (13.0691, 22.8361)
  spline S6 degree 5 poles (13.0691, 22.8361) (13.0745, 22.8455) (13.085, 22.8643) (13.1, 22.893) (13.1188, 22.9319) (13.1404, 22.9814) (13.1608, 23.0315) (13.1803, 23.0821) (13.1994, 23.133) (13.2182, 23.1839) (13.2367, 23.2351) (13.2548, 23.2864) (13.2724, 23.338) (13.2894, 23.3899) (13.3057, 23.4421) (13.3214, 23.4946) (13.3366, 23.5473) (13.3514, 23.6002) (13.3658, 23.6533) (13.3798, 23.7066) (13.3935, 23.76) (13.4069, 23.8135) (13.4198, 23.8673) (13.4324, 23.9212) (13.4445, 23.9753) (13.4563, 24.0295) (13.4677, 24.0839) (13.4788, 24.1385) (13.4895, 24.1932) (13.4999, 24.248) (13.51, 24.3029) (13.5197, 24.358) (13.5291, 24.4132) (13.5382, 24.4686) (13.547, 24.524) (13.5555, 24.5796) (13.5636, 24.6353) (13.5714, 24.6912) (13.579, 24.7471) (13.5862, 24.8032) (13.5932, 24.8593) (13.5998, 24.9156) (13.6062, 24.972) (13.6123, 25.0284) (13.618, 25.085) (13.6235, 25.1417) (13.6288, 25.1985) (13.6337, 25.2553) (13.6383, 25.3123) (13.6427, 25.3694) (13.6468, 25.4265) (13.6507, 25.4838) (13.6542, 25.5411) (13.6575, 25.5985) (13.6606, 25.656) (13.6633, 25.7136) (13.6659, 25.7712) (13.6681, 25.829) (13.6701, 25.8868) (13.6718, 25.9447) (13.6733, 26.0027) (13.6745, 26.0607) (13.6754, 26.1188) (13.6761, 26.177) (13.6766, 26.2353) (13.6768, 26.2936) (13.6767, 26.3521) (13.6765, 26.4105) (13.6759, 26.4691) (13.6751, 26.5277) (13.6741, 26.5863) (13.6731, 26.6333) (13.6722, 26.6686) (13.6715, 26.6921) (13.6712, 26.7039) knots 0 0 0 0 0 0 0.01428571 0.02857143 0.04285714 0.05714286 0.07142857 0.08571429 0.1 0.11428571 0.12857143 0.14285714 0.15714286 0.17142857 0.18571429 0.2 0.21428571 0.22857143 0.24285714 0.25714286 0.27142857 0.28571429 0.3 0.31428571 0.32857143 0.34285714 0.35714286 0.37142857 0.38571429 0.4 0.41428571 0.42857143 0.44285714 0.45714286 0.47142857 0.48571429 0.5 0.51428571 0.52857143 0.54285714 0.55714286 0.57142857 0.58571429 0.6 0.61428571 0.62857143 0.64285714 0.65714286 0.67142857 0.68571429 0.7 0.71428571 0.72857143 0.74285714 0.75714286 0.77142857 0.78571429 0.8 0.81428571 0.82857143 0.84285714 0.85714286 0.87142857 0.88571429 0.9 0.91428571 0.92857143 0.94285714 0.95714286 0.97142857 0.98571429 1 1 1 1 1 1
  arc A8 (13.6712, 26.7039) -> (12.3541, 27.3382) centre (0, 0) ccw
  spline S7 degree 5 poles (9.7055, 24.4559) (9.7095, 24.466) (9.7177, 24.4859) (9.7307, 24.5156) (9.7494, 24.5545) (9.7746, 24.6023) (9.8012, 24.6494) (9.8286, 24.6963) (9.8564, 24.7429) (9.8845, 24.7894) (9.9129, 24.8357) (9.9418, 24.8819) (9.9712, 24.9278) (10.0012, 24.9734) (10.0318, 25.0187) (10.0631, 25.0637) (10.0948, 25.1085) (10.127, 25.153) (10.1595, 25.1974) (10.1924, 25.2416) (10.2256, 25.2856) (10.2591, 25.3294) (10.2931, 25.3731) (10.3274, 25.4165) (10.3621, 25.4597) (10.3972, 25.5027) (10.4326, 25.5456) (10.4683, 25.5882) (10.5044, 25.6307) (10.5408, 25.673) (10.5775, 25.7151) (10.6145, 25.7571) (10.6518, 25.7989) (10.6894, 25.8405) (10.7273, 25.882) (10.7654, 25.9232) (10.8039, 25.9643) (10.8427, 26.0053) (10.8817, 26.0461) (10.921, 26.0867) (10.9606, 26.1271) (11.0004, 26.1674) (11.0406, 26.2075) (11.0809, 26.2475) (11.1216, 26.2873) (11.1624, 26.3269) (11.2036, 26.3664) (11.245, 26.4057) (11.2866, 26.4449) (11.3285, 26.4839) (11.3706, 26.5227) (11.4129, 26.5614) (11.4555, 26.5999) (11.4984, 26.6383) (11.5414, 26.6765) (11.5847, 26.7146) (11.6282, 26.7525) (11.672, 26.7902) (11.716, 26.8279) (11.7601, 26.8653) (11.8046, 26.9026) (11.8492, 26.9397) (11.894, 26.9767) (11.9391, 27.0136) (11.9844, 27.0502) (12.0299, 27.0868) (12.0755, 27.1231) (12.1215, 27.1594) (12.1676, 27.1954) (12.2139, 27.2314) (12.2604, 27.2671) (12.2978, 27.2956) (12.3259, 27.3169) (12.3447, 27.3311) (12.3541, 27.3382) knots 0 0 0 0 0 0 0.01428571 0.02857143 0.04285714 0.05714286 0.07142857 0.08571429 0.1 0.11428571 0.12857143 0.14285714 0.15714286 0.17142857 0.18571429 0.2 0.21428571 0.22857143 0.24285714 0.25714286 0.27142857 0.28571429 0.3 0.31428571 0.32857143 0.34285714 0.35714286 0.37142857 0.38571429 0.4 0.41428571 0.42857143 0.44285714 0.45714286 0.47142857 0.48571429 0.5 0.51428571 0.52857143 0.54285714 0.55714286 0.57142857 0.58571429 0.6 0.61428571 0.62857143 0.64285714 0.65714286 0.67142857 0.68571429 0.7 0.71428571 0.72857143 0.74285714 0.75714286 0.77142857 0.78571429 0.8 0.81428571 0.82857143 0.84285714 0.85714286 0.87142857 0.88571429 0.9 0.91428571 0.92857143 0.94285714 0.95714286 0.97142857 0.98571429 1 1 1 1 1 1
  line L7 (9.7055, 24.4559) -> (9.4748, 23.8746)
  arc A9 (9.4748, 23.8746) -> (7.4779, 24.5734) centre (0, 0) ccw
  line L8 (7.4779, 24.5734) -> (7.6599, 25.1717)
  spline S8 degree 5 poles (7.6599, 25.1717) (7.6631, 25.182) (7.6691, 25.2028) (7.6774, 25.2341) (7.6871, 25.2761) (7.6971, 25.3292) (7.7058, 25.3826) (7.7136, 25.4363) (7.7209, 25.4901) (7.7279, 25.544) (7.7346, 25.598) (7.7408, 25.6521) (7.7465, 25.7063) (7.7514, 25.7606) (7.7557, 25.8152) (7.7594, 25.8698) (7.7625, 25.9246) (7.7651, 25.9795) (7.7673, 26.0345) (7.7692, 26.0895) (7.7706, 26.1446) (7.7717, 26.1998) (7.7724, 26.2551) (7.7726, 26.3104) (7.7725, 26.3659) (7.7719, 26.4214) (7.7709, 26.4769) (7.7695, 26.5326) (7.7678, 26.5883) (7.7657, 26.644) (7.7633, 26.6999) (7.7606, 26.7557) (7.7575, 26.8117) (7.754, 26.8676) (7.7502, 26.9237) (7.7461, 26.9797) (7.7417, 27.0359) (7.7369, 27.092) (7.7318, 27.1483) (7.7264, 27.2045) (7.7206, 27.2608) (7.7146, 27.3172) (7.7083, 27.3735) (7.7016, 27.4299) (7.6947, 27.4864) (7.6874, 27.5429) (7.6799, 27.5994) (7.672, 27.6559) (7.6639, 27.7125) (7.6555, 27.7691) (7.6468, 27.8257) (7.6378, 27.8824) (7.6285, 27.9391) (7.6189, 27.9958) (7.6091, 28.0525) (7.599, 28.1093) (7.5886, 28.166) (7.5779, 28.2228) (7.567, 28.2796) (7.5558, 28.3365) (7.5443, 28.3933) (7.5326, 28.4502) (7.5206, 28.5071) (7.5083, 28.564) (7.4958, 28.6209) (7.483, 28.6778) (7.47, 28.7347) (7.4567, 28.7917) (7.4431, 28.8486) (7.4293, 28.9056) (7.4152, 28.9625) (7.4038, 29.0081) (7.3951, 29.0423) (7.3892, 29.0651) (7.3863, 29.0765) knots 0 0 0 0 0 0 0.01428571 0.02857143 0.04285714 0.05714286 0.07142857 0.08571429 0.1 0.11428571 0.12857143 0.14285714 0.15714286 0.17142857 0.18571429 0.2 0.21428571 0.22857143 0.24285714 0.25714286 0.27142857 0.28571429 0.3 0.31428571 0.32857143 0.34285714 0.35714286 0.37142857 0.38571429 0.4 0.41428571 0.42857143 0.44285714 0.45714286 0.47142857 0.48571429 0.5 0.51428571 0.52857143 0.54285714 0.55714286 0.57142857 0.58571429 0.6 0.61428571 0.62857143 0.64285714 0.65714286 0.67142857 0.68571429 0.7 0.71428571 0.72857143 0.74285714 0.75714286 0.77142857 0.78571429 0.8 0.81428571 0.82857143 0.84285714 0.85714286 0.87142857 0.88571429 0.9 0.91428571 0.92857143 0.94285714 0.95714286 0.97142857 0.98571429 1 1 1 1 1 1
  arc A10 (7.3863, 29.0765) -> (5.961, 29.4018) centre (0, 0) ccw
  spline S9 degree 5 poles (4.0202, 26.0024) (4.0219, 26.0131) (4.0254, 26.0344) (4.0315, 26.0662) (4.0411, 26.1083) (4.055, 26.1605) (4.0704, 26.2124) (4.0867, 26.2641) (4.1034, 26.3158) (4.1205, 26.3674) (4.1379, 26.4189) (4.1558, 26.4703) (4.1742, 26.5216) (4.1933, 26.5728) (4.2131, 26.6237) (4.2336, 26.6746) (4.2545, 26.7253) (4.276, 26.7759) (4.2978, 26.8263) (4.32, 26.8767) (4.3426, 26.927) (4.3656, 26.9772) (4.389, 27.0273) (4.4128, 27.0773) (4.437, 27.1272) (4.4616, 27.1769) (4.4866, 27.2266) (4.512, 27.2761) (4.5377, 27.3255) (4.5637, 27.3749) (4.5901, 27.4241) (4.6168, 27.4733) (4.6439, 27.5223) (4.6713, 27.5712) (4.699, 27.6201) (4.7271, 27.6688) (4.7554, 27.7175) (4.7841, 27.766) (4.8131, 27.8144) (4.8424, 27.8628) (4.872, 27.911) (4.9018, 27.9591) (4.932, 28.0072) (4.9625, 28.0551) (4.9932, 28.103) (5.0243, 28.1507) (5.0556, 28.1983) (5.0872, 28.2459) (5.1191, 28.2933) (5.1512, 28.3407) (5.1836, 28.3879) (5.2163, 28.4351) (5.2493, 28.4821) (5.2825, 28.529) (5.316, 28.5759) (5.3497, 28.6226) (5.3837, 28.6693) (5.418, 28.7158) (5.4525, 28.7623) (5.4872, 28.8086) (5.5222, 28.8548) (5.5574, 28.901) (5.5929, 28.947) (5.6287, 28.993) (5.6647, 29.0388) (5.7009, 29.0845) (5.7373, 29.1302) (5.774, 29.1757) (5.8109, 29.2211) (5.8481, 29.2665) (5.8855, 29.3117) (5.9156, 29.3478) (5.9383, 29.3748) (5.9534, 29.3928) (5.961, 29.4018) knots 0 0 0 0 0 0 0.01428571 0.02857143 0.04285714 0.05714286 0.07142857 0.08571429 0.1 0.11428571 0.12857143 0.14285714 0.15714286 0.17142857 0.18571429 0.2 0.21428571 0.22857143 0.24285714 0.25714286 0.27142857 0.28571429 0.3 0.31428571 0.32857143 0.34285714 0.35714286 0.37142857 0.38571429 0.4 0.41428571 0.42857143 0.44285714 0.45714286 0.47142857 0.48571429 0.5 0.51428571 0.52857143 0.54285714 0.55714286 0.57142857 0.58571429 0.6 0.61428571 0.62857143 0.64285714 0.65714286 0.67142857 0.68571429 0.7 0.71428571 0.72857143 0.74285714 0.75714286 0.77142857 0.78571429 0.8 0.81428571 0.82857143 0.84285714 0.85714286 0.87142857 0.88571429 0.9 0.91428571 0.92857143 0.94285714 0.95714286 0.97142857 0.98571429 1 1 1 1 1 1
  line L9 (4.0202, 26.0024) -> (3.9247, 25.3844)
  arc A11 (3.9247, 25.3844) -> (1.8223, 25.6213) centre (0, 0) ccw
  line L10 (1.8223, 25.6213) -> (1.8667, 26.2451)
  spline S10 degree 5 poles (1.8667, 26.2451) (1.8674, 26.2559) (1.8687, 26.2774) (1.8698, 26.3098) (1.8699, 26.3529) (1.8679, 26.4069) (1.8644, 26.461) (1.8601, 26.515) (1.8552, 26.5691) (1.8501, 26.6232) (1.8446, 26.6773) (1.8386, 26.7314) (1.8321, 26.7855) (1.8248, 26.8396) (1.8169, 26.8937) (1.8082, 26.9478) (1.7991, 27.0019) (1.7894, 27.056) (1.7794, 27.1101) (1.7689, 27.1642) (1.7581, 27.2182) (1.7469, 27.2723) (1.7352, 27.3263) (1.7231, 27.3803) (1.7106, 27.4343) (1.6977, 27.4883) (1.6844, 27.5423) (1.6707, 27.5962) (1.6566, 27.6502) (1.6422, 27.7041) (1.6274, 27.7579) (1.6123, 27.8118) (1.5968, 27.8656) (1.581, 27.9194) (1.5648, 27.9732) (1.5483, 28.027) (1.5315, 28.0807) (1.5143, 28.1344) (1.4969, 28.1881) (1.4791, 28.2417) (1.461, 28.2953) (1.4425, 28.3489) (1.4238, 28.4025) (1.4048, 28.456) (1.3854, 28.5095) (1.3658, 28.5629) (1.3459, 28.6163) (1.3256, 28.6697) (1.3051, 28.7231) (1.2843, 28.7764) (1.2632, 28.8296) (1.2418, 28.8829) (1.2202, 28.9361) (1.1983, 28.9892) (1.176, 29.0423) (1.1536, 29.0954) (1.1308, 29.1485) (1.1078, 29.2015) (1.0845, 29.2544) (1.0609, 29.3073) (1.0371, 29.3602) (1.013, 29.413) (0.9886, 29.4658) (0.964, 29.5186) (0.9391, 29.5712) (0.914, 29.6239) (0.8886, 29.6765) (0.863, 29.729) (0.8371, 29.7816) (0.8109, 29.834) (0.7845, 29.8864) (0.7632, 29.9283) (0.7471, 29.9597) (0.7364, 29.9806) (0.731, 29.9911) knots 0 0 0 0 0 0 0.01428571 0.02857143 0.04285714 0.05714286 0.07142857 0.08571429 0.1 0.11428571 0.12857143 0.14285714 0.15714286 0.17142857 0.18571429 0.2 0.21428571 0.22857143 0.24285714 0.25714286 0.27142857 0.28571429 0.3 0.31428571 0.32857143 0.34285714 0.35714286 0.37142857 0.38571429 0.4 0.41428571 0.42857143 0.44285714 0.45714286 0.47142857 0.48571429 0.5 0.51428571 0.52857143 0.54285714 0.55714286 0.57142857 0.58571429 0.6 0.61428571 0.62857143 0.64285714 0.65714286 0.67142857 0.68571429 0.7 0.71428571 0.72857143 0.74285714 0.75714286 0.77142857 0.78571429 0.8 0.81428571 0.82857143 0.84285714 0.85714286 0.87142857 0.88571429 0.9 0.91428571 0.92857143 0.94285714 0.95714286 0.97142857 0.98571429 1 1 1 1 1 1
  arc A12 (0.731, 29.9911) -> (-0.731, 29.9911) centre (0, 0) ccw
  spline S11 degree 5 poles (-1.8667, 26.2451) (-1.8674, 26.2559) (-1.8687, 26.2774) (-1.8698, 26.3098) (-1.8699, 26.3529) (-1.8679, 26.4069) (-1.8644, 26.461) (-1.8601, 26.515) (-1.8552, 26.5691) (-1.8501, 26.6232) (-1.8446, 26.6773) (-1.8386, 26.7314) (-1.8321, 26.7855) (-1.8248, 26.8396) (-1.8169, 26.8937) (-1.8082, 26.9478) (-1.7991, 27.0019) (-1.7894, 27.056) (-1.7794, 27.1101) (-1.7689, 27.1642) (-1.7581, 27.2182) (-1.7469, 27.2723) (-1.7352, 27.3263) (-1.7231, 27.3803) (-1.7106, 27.4343) (-1.6977, 27.4883) (-1.6844, 27.5423) (-1.6707, 27.5962) (-1.6566, 27.6502) (-1.6422, 27.7041) (-1.6274, 27.7579) (-1.6123, 27.8118) (-1.5968, 27.8656) (-1.581, 27.9194) (-1.5648, 27.9732) (-1.5483, 28.027) (-1.5315, 28.0807) (-1.5143, 28.1344) (-1.4969, 28.1881) (-1.4791, 28.2417) (-1.461, 28.2953) (-1.4425, 28.3489) (-1.4238, 28.4025) (-1.4048, 28.456) (-1.3854, 28.5095) (-1.3658, 28.5629) (-1.3459, 28.6163) (-1.3256, 28.6697) (-1.3051, 28.7231) (-1.2843, 28.7764) (-1.2632, 28.8296) (-1.2418, 28.8829) (-1.2202, 28.9361) (-1.1983, 28.9892) (-1.176, 29.0423) (-1.1536, 29.0954) (-1.1308, 29.1485) (-1.1078, 29.2015) (-1.0845, 29.2544) (-1.0609, 29.3073) (-1.0371, 29.3602) (-1.013, 29.413) (-0.9886, 29.4658) (-0.964, 29.5186) (-0.9391, 29.5712) (-0.914, 29.6239) (-0.8886, 29.6765) (-0.863, 29.729) (-0.8371, 29.7816) (-0.8109, 29.834) (-0.7845, 29.8864) (-0.7632, 29.9283) (-0.7471, 29.9597) (-0.7364, 29.9806) (-0.731, 29.9911) knots 0 0 0 0 0 0 0.01428571 0.02857143 0.04285714 0.05714286 0.07142857 0.08571429 0.1 0.11428571 0.12857143 0.14285714 0.15714286 0.17142857 0.18571429 0.2 0.21428571 0.22857143 0.24285714 0.25714286 0.27142857 0.28571429 0.3 0.31428571 0.32857143 0.34285714 0.35714286 0.37142857 0.38571429 0.4 0.41428571 0.42857143 0.44285714 0.45714286 0.47142857 0.48571429 0.5 0.51428571 0.52857143 0.54285714 0.55714286 0.57142857 0.58571429 0.6 0.61428571 0.62857143 0.64285714 0.65714286 0.67142857 0.68571429 0.7 0.71428571 0.72857143 0.74285714 0.75714286 0.77142857 0.78571429 0.8 0.81428571 0.82857143 0.84285714 0.85714286 0.87142857 0.88571429 0.9 0.91428571 0.92857143 0.94285714 0.95714286 0.97142857 0.98571429 1 1 1 1 1 1
  line L11 (-1.8667, 26.2451) -> (-1.8223, 25.6213)
  arc A13 (-1.8223, 25.6213) -> (-3.9247, 25.3844) centre (0, 0) ccw
  line L12 (-3.9247, 25.3844) -> (-4.0202, 26.0024)
  spline S12 degree 5 poles (-4.0202, 26.0024) (-4.0219, 26.0131) (-4.0254, 26.0344) (-4.0315, 26.0662) (-4.0411, 26.1083) (-4.055, 26.1605) (-4.0704, 26.2124) (-4.0867, 26.2641) (-4.1034, 26.3158) (-4.1205, 26.3674) (-4.1379, 26.4189) (-4.1558, 26.4703) (-4.1742, 26.5216) (-4.1933, 26.5728) (-4.2131, 26.6237) (-4.2336, 26.6746) (-4.2545, 26.7253) (-4.276, 26.7759) (-4.2978, 26.8263) (-4.32, 26.8767) (-4.3426, 26.927) (-4.3656, 26.9772) (-4.389, 27.0273) (-4.4128, 27.0773) (-4.437, 27.1272) (-4.4616, 27.1769) (-4.4866, 27.2266) (-4.512, 27.2761) (-4.5377, 27.3255) (-4.5637, 27.3749) (-4.5901, 27.4241) (-4.6168, 27.4733) (-4.6439, 27.5223) (-4.6713, 27.5712) (-4.699, 27.6201) (-4.7271, 27.6688) (-4.7554, 27.7175) (-4.7841, 27.766) (-4.8131, 27.8144) (-4.8424, 27.8628) (-4.872, 27.911) (-4.9018, 27.9591) (-4.932, 28.0072) (-4.9625, 28.0551) (-4.9932, 28.103) (-5.0243, 28.1507) (-5.0556, 28.1983) (-5.0872, 28.2459) (-5.1191, 28.2933) (-5.1512, 28.3407) (-5.1836, 28.3879) (-5.2163, 28.4351) (-5.2493, 28.4821) (-5.2825, 28.529) (-5.316, 28.5759) (-5.3497, 28.6226) (-5.3837, 28.6693) (-5.418, 28.7158) (-5.4525, 28.7623) (-5.4872, 28.8086) (-5.5222, 28.8548) (-5.5574, 28.901) (-5.5929, 28.947) (-5.6287, 28.993) (-5.6647, 29.0388) (-5.7009, 29.0845) (-5.7373, 29.1302) (-5.774, 29.1757) (-5.8109, 29.2211) (-5.8481, 29.2665) (-5.8855, 29.3117) (-5.9156, 29.3478) (-5.9383, 29.3748) (-5.9534, 29.3928) (-5.961, 29.4018) knots 0 0 0 0 0 0 0.01428571 0.02857143 0.04285714 0.05714286 0.07142857 0.08571429 0.1 0.11428571 0.12857143 0.14285714 0.15714286 0.17142857 0.18571429 0.2 0.21428571 0.22857143 0.24285714 0.25714286 0.27142857 0.28571429 0.3 0.31428571 0.32857143 0.34285714 0.35714286 0.37142857 0.38571429 0.4 0.41428571 0.42857143 0.44285714 0.45714286 0.47142857 0.48571429 0.5 0.51428571 0.52857143 0.54285714 0.55714286 0.57142857 0.58571429 0.6 0.61428571 0.62857143 0.64285714 0.65714286 0.67142857 0.68571429 0.7 0.71428571 0.72857143 0.74285714 0.75714286 0.77142857 0.78571429 0.8 0.81428571 0.82857143 0.84285714 0.85714286 0.87142857 0.88571429 0.9 0.91428571 0.92857143 0.94285714 0.95714286 0.97142857 0.98571429 1 1 1 1 1 1
  arc A14 (-5.961, 29.4018) -> (-7.3863, 29.0765) centre (0, 0) ccw